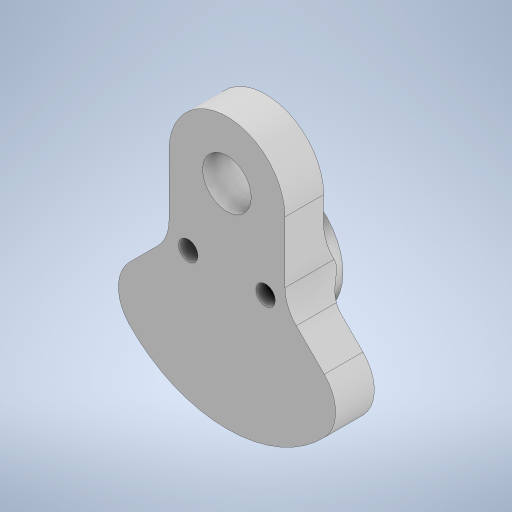
# Autodesk Inventor part: Crank on Crankshaft
Saved by Autodesk Inventor 2023 (Build 270158000, 158)
## iProperties
Created: 2022-10-29
Part Number: Crank on Crankshaft
Material: Generic
Document SubType Name: Modeling
Designer: tommy
Density: 1 g/cm^3
Appearance: Default
Author: tommy
Autodesk Inventor part; units mm, degrees
ref_plane "YZ Plane" through (0, 0, 0) normal (1, 0, 0) x (0, 1, 0)
ref_plane "XZ Plane" through (0, 0, 0) normal (0, 1, 0) x (-1, 0, 0)
ref_plane "XY Plane" through (0, 0, 0) normal (0, 0, 1) x (1, 0, 0)
sketch "Sketch1" plane through (0, 0, 0) normal (0, 0, 1) x (1, 0, 0)
  circle A0 centre (0, 12.7) radius 3.9878
  line L0 (-11.3849, -1.8599) -> (-13.7386, -4.2136)
  line L1 (11.3849, -1.8599) -> (13.7386, -4.2136)
  circle A1 centre (-6.35, 0) radius 1.5875
  circle A2 centre (6.35, 0) radius 1.5875
  line L2 (-9.525, 2.6303) -> (-9.525, 12.7)
  line L3 (9.525, 2.6303) -> (9.525, 12.7)
  arc A3 (9.525, 12.7) -> (-9.525, 12.7) centre (0, 12.7) ccw
  arc A4 (9.525, 12.7) -> (-9.525, 12.7) centre (0, 12.7) ccw
  arc A5 (-16.0921, -15.3295) -> (16.0921, -15.3295) centre (0, 0) ccw
  line L4 (-11.3849, -1.8599) -> (-15.9845, -6.4595)
  line L5 (11.3849, -1.8599) -> (15.9845, -6.4595)
  arc A6 (-15.9845, -6.4595) -> (-16.0921, -15.3295) centre (-11.4944, -10.9496) ccw
  arc A7 (16.0921, -15.3295) -> (15.9845, -6.4595) centre (11.4944, -10.9496) ccw
  arc A8 (-11.3849, -1.8599) -> (-9.525, 2.6303) centre (-15.875, 2.6303) ccw
  arc A9 (9.525, 2.6303) -> (11.3849, -1.8599) centre (15.875, 2.6303) ccw
  arc A10 (-4.6113, 8.3344) -> (4.6113, 8.3344) centre (0, 12.7) ccw
  arc A11 (-4.6113, 8.3344) -> (4.6113, 8.3344) centre (0, 0) ccw
  point P0 (0, 19.05)
  point P1 (-9.525, 0)
  point P2 (-17.3629, -7.8379)
  point P3 (9.525, 0)
  point P4 (17.3629, -7.8379)
  point P5 (-19.7389, -10.2139)
  point P6 (19.7389, -10.2139)
  dimension "d20" = 7.9756
  dimension "d34" = 44.45
  dimension "d35" = 6.35
  dimension "d36" = 6.35
  dimension "d38" = 12.7
  constraints: 20 point on circle, 12 centre point, 12 end point, 9 tangent, 8 point on line, 4 coincident, 2 equal radius, 1 parallel, 1 vertical
  measures "d20" diameter of A0
  measures "d34" diameter of A5
  measures "d35" radius of A6
  measures "d36" radius of A8
  measures "d38" diameter of A10
extrude "Extrusion2" add sketch "Sketch1" along normal blind 6.35 contours A8 L2 A3 L3 A9 L1 L5 A7 A5 A6 L4 L0 | A10 A11
extrude "Extrusion3" add sketch "Sketch1" against normal blind 3.175 contours A10 A11
fillet "Fillet1" radius 3.175 1 edges at (0, -9.525, 0)
body "Solid2"
